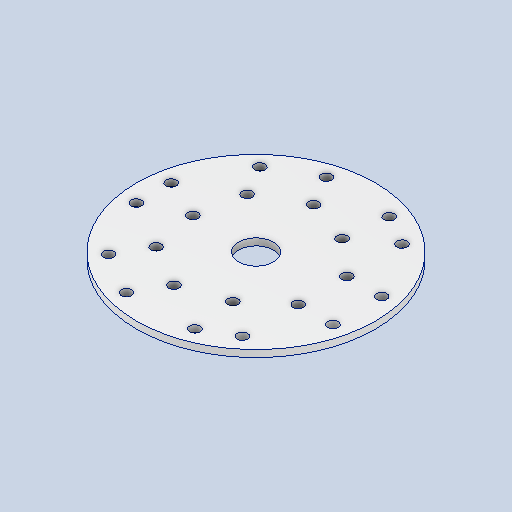
# Autodesk Inventor part: hand-grab-v1-MDF-air-Base
Saved by Autodesk Inventor 2025.1 (Build 291241000, 241)
## iProperties
Created: 2024-10-07
Part Number: hand-grab-v1-MDF-air-Base
Material: アルミニウム 6061
Document SubType Name: Modeling
Designer: haruy
Density: 2.7 g/cm^3
Appearance: アルミニウム - フラット
Author: haruy
Autodesk Inventor part; units mm, degrees
ref_plane "YZ Plane" through (0, 0, 0) normal (1, 0, 0) x (0, 1, 0)
ref_plane "XZ Plane" through (0, 0, 0) normal (0, 1, 0) x (-1, 0, 0)
ref_plane "XY Plane" through (0, 0, 0) normal (0, 0, 1) x (1, 0, 0)
derived "hand-grab-v1-Sketch-Base.ipt"
sketch "スケッチ1" plane through (400, 0, 0) normal (1, 0, 0) x (0, 1, 0)
  circle A0 centre (0, 0) radius 120
  circle A1 centre (-109.5522, 63.25) radius 6.5
  line L0 (0, 0) -> (-109.5522, 63.25)
  line L1 (0, 0) -> (0, 120)
  line L2 (246.0862, 200) -> (-251.4603, 200)
  circle A2 centre (145, 60) radius 254.573
  circle A3 centre (-67.6203, 200) radius 6.5
  line L3 (0, 0) -> (-120, 0)
  line L4 (249, 9.15) -> (187, 9.15)
  line L5 (187, 9.15) -> (187, -9.15)
  line L6 (187, -9.15) -> (249, -9.15)
  line L7 (249, -9.15) -> (249, 9.15)
  line L8 (187, 5.15) -> (179, 5.15)
  line L9 (179, 5.15) -> (179, -4.85)
  line L10 (179, -4.85) -> (187, -4.85)
  line L11 (187, -4.85) -> (187, 5.15)
  line L12 (179, 3.15) -> (174, 3.15)
  line L13 (174, 3.15) -> (174, -2.85)
  line L14 (174, -2.85) -> (179, -2.85)
  line L15 (179, -2.85) -> (179, 3.15)
  line L16 (174, 2.65) -> (159, 2.65)
  line L17 (159, 2.65) -> (159, -2.35)
  line L18 (159, -2.35) -> (174, -2.35)
  line L19 (174, -2.35) -> (174, 2.65)
  line L20 (187, 34.15) -> (184, 34.15)
  line L21 (184, 34.15) -> (184, -43.5182)
  line L22 (184, -43.5182) -> (187, -43.5182)
  line L23 (187, -43.5182) -> (187, 34.15)
  circle A4 centre (150, 65) radius 4
  circle A5 centre (150, 65) radius 14
  line L24 (187, 34.15) -> (192, 34.15)
  line L25 (192, 34.15) -> (192, 14.15)
  line L26 (192, 14.15) -> (187, 14.15)
  line L27 (187, 14.15) -> (187, 34.15)
  line L28 (184, 34.15) -> (147.5804, 61.8148)
  line L29 (151.3533, 68.7641) -> (192, 54.15)
  line L30 (192, 54.15) -> (192, 34.15)
  line L31 (239.3868, 130) -> (-239.3868, 130)
  circle A6 centre (-109.5522, 63.25) radius 4
  circle A7 centre (150, 65) radius 9
  line L32 (-106.0881, 61.25) -> (-113.0163, 65.25)
  line L33 (170, 36) -> (155, 36)
  circle A8 centre (155, 36) radius 5
  circle A9 centre (155, 36) radius 9
  circle A10 centre (-90.698, 156.1969) radius 6.5
  circle A11 centre (170, 36) radius 5
  line L34 (150, 65) -> (170, 36)
  circle A12 centre (170, 36) radius 9
  circle A13 centre (150, 65) radius 44.2278
  line L35 (150, 65) -> (155, 36)
  line L36 (150, 65) -> (-109.5522, 63.25)
  line L37 (-90.698, 156.1969) -> (150, 65)
  line L38 (150, 65) -> (157.5146, 21.4152)
  circle A14 centre (150, 65) radius 35.2278
  circle A15 centre (155.9855, 30.2844) radius 9
  line L39 (168.0777, 21.2844) -> (136, 21.2844)
  line L40 (175, 3.15) -> (175, -2.85)
  point P0 (-60, 0)
sketch "スケッチ2" plane through (0, 400, 0) normal (0, 1, 0) x (-1, 0, 0)
  circle A0 centre (0, 0) radius 120
  line L0 (0, 0) -> (-331.4625, 0) construction
  line L1 (67.5, -116.9134) -> (-135, 0)
  circle A1 centre (0, 0) radius 5
  line L2 (0, 0) -> (67.5, 116.9134) construction
  line L3 (0, 0) -> (67.5, -116.9134) construction
  line L4 (0, 0) -> (-135, 0)
  line L5 (17.0359, 37.507) -> (12.0359, 28.8468) construction
  line L6 (12.0359, 28.8468) -> (15.5, 26.8468) construction
  line L7 (15.5, 26.8468) -> (20.5, 35.507) construction
  line L8 (20.5, 35.507) -> (17.0359, 37.507)
  line L9 (20.5, 35.507) -> (15.5, 26.8468) construction
  line L10 (15.5, 26.8468) -> (18.9641, 24.8468) construction
  line L11 (18.9641, 24.8468) -> (23.9641, 33.507) construction
  line L12 (23.9641, 33.507) -> (20.5, 35.507)
  line L13 (14.5359, 33.1769) -> (21.4641, 29.1769) construction
  circle A2 centre (0, 0) radius 2.65 construction
  line L14 (16.8194, 37.632) -> (10.3194, 26.3737) construction
  line L15 (10.3194, 26.3737) -> (5.9893, 28.8737) construction
  line L16 (5.9893, 28.8737) -> (12.4893, 40.132) construction
  line L17 (12.4893, 40.132) -> (16.8194, 37.632)
  line L18 (28.5107, 30.882) -> (24.1806, 33.382)
  line L19 (22.0107, 19.6237) -> (28.5107, 30.882) construction
  line L20 (24.1806, 33.382) -> (17.6806, 22.1237) construction
  line L21 (17.6806, 22.1237) -> (22.0107, 19.6237) construction
  circle A3 centre (0, 0) radius 28.3207 construction
  line L22 (-41, 9.25) -> (-41, 4.25)
  line L23 (-41, 4.25) -> (-28, 4.25) construction
  line L24 (-28, 9.25) -> (-41, 9.25) construction
  line L25 (-28, 4.25) -> (-28, 9.25)
  line L26 (-41, -4.25) -> (-28, -4.25) construction
  line L27 (-41, -9.25) -> (-41, -4.25)
  line L28 (-28, -9.25) -> (-41, -9.25) construction
  line L29 (-28, -4.25) -> (-28, -9.25)
  line L30 (12.4893, -40.132) -> (16.8194, -37.632)
  line L31 (16.8194, -37.632) -> (10.3194, -26.3737) construction
  line L32 (5.9893, -28.8737) -> (12.4893, -40.132) construction
  line L33 (10.3194, -26.3737) -> (5.9893, -28.8737) construction
  line L34 (24.1806, -33.382) -> (17.6806, -22.1237) construction
  line L35 (28.5107, -30.882) -> (24.1806, -33.382)
  line L36 (22.0107, -19.6237) -> (28.5107, -30.882) construction
  line L37 (17.6806, -22.1237) -> (22.0107, -19.6237) construction
  line L38 (5.9893, 28.8737) -> (5.373, 27.8064)
  line L39 (22.0107, 19.6237) -> (21.3945, 18.5564) construction
  line L40 (-28, 9.25) -> (-26.7675, 9.25)
  line L41 (-28, -9.25) -> (-26.7675, -9.25)
  line L42 (5.9893, -28.8737) -> (2.1934, -22.2991) construction
  line L43 (22.0107, -19.6237) -> (21.3945, -18.5564) construction
  line L44 (13.6109, 31.5748) -> (3.6109, 14.2543) construction
  line L45 (3.6109, 14.2543) -> (-1.5853, 17.2543) construction
  line L46 (-1.5853, 17.2543) -> (8.4147, 34.5748) construction
  line L47 (8.4147, 34.5748) -> (13.6109, 31.5748)
  circle A4 centre (3.5128, 20.0844) radius 1.5
  circle A5 centre (8.5128, 28.7446) radius 1.5
  circle A6 centre (20.6372, 21.7446) radius 1.5
  circle A7 centre (15.6372, 13.0844) radius 1.5
  circle A8 centre (-29.15, 7) radius 1.5
  circle A9 centre (-19.15, 7) radius 1.5
  circle A10 centre (-19.15, -7) radius 1.5
  circle A11 centre (-29.15, -7) radius 1.5
  circle A12 centre (8.5128, -28.7446) radius 1.5
  circle A13 centre (3.5128, -20.0844) radius 1.5
  circle A14 centre (15.6372, -13.0844) radius 1.5
  circle A15 centre (20.6372, -21.7446) radius 1.5
  line L48 (1.0128, 15.7543) -> (13.6109, 31.5748) construction
  circle A16 centre (0, 0) radius 34.3835
  line L49 (-8, 47) -> (-188, 47) construction
  line L50 (-188, 47) -> (-188, 32)
  line L51 (-188, 32) -> (-8, 32) construction
  line L52 (-8, 32) -> (-8, 47) construction
  circle A17 centre (-18, 39.5) radius 1.5 construction
  circle A18 centre (-28, 39.5) radius 1.5 construction
  line L53 (-34.3835, 47) -> (-34.3835, 0) construction
  line L54 (-8, 47) -> (19.3201, 28.4422) construction
  line L55 (-8, -47) -> (-188, -47) construction
  line L56 (-188, -32) -> (-8, -32) construction
  circle A19 centre (-18, -39.5) radius 1.5 construction
  circle A20 centre (-28, -39.5) radius 1.5 construction
  line L57 (-34.3835, -47) -> (-34.3835, 0) construction
  line L58 (-8, -47) -> (19.3201, -28.4422) construction
  line L59 (0, 0) -> (-17.1917, 29.777)
  line L60 (-8.5315, 34.777) -> (-25.852, 24.777)
  line L61 (-25.852, 24.777) -> (-20.852, 16.1167)
  line L62 (-20.852, 16.1167) -> (-3.5315, 26.1167)
  line L63 (-3.5315, 26.1167) -> (-8.5315, 34.777)
  circle A21 centre (-10.3616, 27.9468) radius 1.5
  circle A22 centre (-19.0219, 22.9468) radius 1.5
  circle A23 centre (-19.0219, -22.9468) radius 1.5
  circle A24 centre (-10.3616, -27.9468) radius 1.5
  circle A25 centre (29.3835, -5) radius 1.5
  circle A26 centre (29.3835, 5) radius 1.5
  circle A27 centre (0, 0) radius 193.5
  line L64 (-192.8647, 15.6665) -> (82.8647, 174.859)
  line L65 (0, 0) -> (-60, 103.923)
  line L66 (0, 0) -> (0, 193.5)
  line L67 (53.3013, 7.6795) -> (-48.1987, 183.4826)
  line L68 (-48.1987, 183.4826) -> (-61.1891, 175.9826)
  line L69 (-61.1891, 175.9826) -> (40.3109, 0.1795)
  line L70 (40.3109, 0.1795) -> (53.3013, 7.6795)
  circle A28 centre (-21.9439, 123.008) radius 1.5
  circle A29 centre (-50.9439, 173.2375) radius 1.5
  circle A30 centre (-9.0667, 15.704) radius 1.5
  circle A31 centre (0, 0) radius 12.5
  circle A32 centre (-9.0667, -15.704) radius 1.5
  circle A33 centre (18.1335, 0) radius 1.5
  circle A34 centre (41.8061, 12.5897) radius 1.5
  circle A35 centre (31.8061, 29.9103) radius 1.5
  circle A36 centre (0, 0) radius 24.3835
  line L71 (53.3013, 7.6795) -> (22.0795, -10.3464)
  line L72 (33.3013, 42.3205) -> (2.0795, 24.2946)
  line L73 (-33.3013, -42.3205) -> (-134.8013, 133.4826)
  line L74 (-20.3109, -34.8205) -> (-33.3013, -42.3205)
  circle A37 centre (-31.8061, -29.9103) radius 1.5
  circle A38 centre (-41.8061, -12.5897) radius 1.5
  line L75 (-33.3013, -42.3205) -> (-2.0795, -24.2946)
  line L76 (-53.3013, -7.6795) -> (-22.0795, 10.3464)
  point P0 (19.3201, -28.4422)
  dimension "d3" = 3
  dimension "d4" = 3
  dimension "d5" = 10
  dimension "d6" = 10
  dimension "d7" = 7.5
  dimension "d8" = 7.5
  dimension "d10" = 60
  dimension "d12" = 10
  dimension "d13" = 10
  dimension "d14" = 10
  dimension "d15" = 3
  dimension "d17" = 5
  dimension "d18" = 5
  dimension "d21" = 360
  dimension "d25" = 387
  dimension "d26" = 110
  dimension "d27" = 60
  dimension "d28" = 15
  dimension "d30" = 73
  dimension "d31" = 3
  dimension "d32" = 3
  dimension "d33" = 7.5
  dimension "d34" = 7.5
  dimension "d35" = 7.5
  dimension "d36" = 7.5
  dimension "d37" = 3
  dimension "d38" = 25
  dimension "d39" = 6.25
  dimension "d42" = 360
  dimension "d44" = 20
  dimension "d45" = 3
  dimension "d46" = 3
  dimension "d47" = 10
  dimension "d48" = 7.5
  dimension "d49" = 7.5
  dimension "d50" = 20
  dimension "d51" = 35
  dimension "d52" = 10
  measures "d3" diameter of A17
  measures "d4" diameter of A18
  measures "d5" distance from line of A17.centre L52
  measures "d6" distance of A18.centre A17.centre
  measures "d7" distance from line of A17.centre L49
  measures "d8" distance from line of L49 A18.centre
  measures "d12" distance between parallel lines of L60 L62
  measures "d13" distance between parallel lines of L63 L59
  measures "d14" distance between parallel lines of L59 L61
  measures "d15" diameter of A21
  measures "d17" distance from line of L59 A21.centre
  measures "d18" distance from line of A21.centre L60
  measures "d25" diameter of A27
  measures "d26" distance from line of L64 A3.centre
  measures "d28" distance of L68.end L67.end
  measures "d30" distance between parallel lines of L64 L68
  measures "d31" diameter of A28
  measures "d32" diameter of A29
  measures "d33" distance from line of A28.centre L64
  measures "d34" distance from line of A28.centre L69
  measures "d35" distance from line of A29.centre L68
  measures "d36" distance from line of A29.centre L67
  measures "d37" diameter of A30
  measures "d38" diameter of A31
  measures "d39" distance from line of A30.centre L62
  measures "d44" distance from line of L70 point (0, 0)
  measures "d45" diameter of A34
  measures "d46" diameter of A35
  measures "d47" distance from line of A34.centre L70
  measures "d48" distance from line of L67 A35.centre
  measures "d49" distance from line of L67 A34.centre
  measures "d50" distance of A35.centre A34.centre
  measures "d51" distance from line of L69 point (0, 0)
  measures "d52" distance from line of L72 A35.centre
ref_plane "作業平面1" through (400, 0, 0) normal (1, 0, 0) x (0, 1, 0)
ref_plane "作業平面2" through (0, 400, 0) normal (0, 1, 0) x (-1, 0, 0)
extrude "押し出し1" add sketch "スケッチ2" along normal blind 2 contours L66 A36 L62 L63 A16 | A16 L72 A5 A36 L66 | L63 L62 L59 A16 | A36 L4 A31 L66 | L66 A31 L59 A30 A36 | L59 L62 L61 A16 | A16 L71 A25 A36 L72 A5 | A31 L4 A1 L66 | L66 A1 L59 A31 | A36 L76 A8 A16 L61 L62 | L59 A30 A31 L4 A36 | A16 L75 A24 A36 L71 A25 | A16 L76 A8 A36 L4 | L4 A36 L75 A24 A16 | L59 A1 L4 A31
sketch "スケッチ3" plane through (0, 402, 0) normal (0, 1, 0) x (0, 0, -1)
  circle A0 centre (0, 0) radius 34.3835 projected
  circle A1 centre (0, 0) radius 5 projected
  circle A2 centre (21.7446, 20.6372) radius 1.5 projected
  circle A3 centre (13.0844, 15.6372) radius 1.5 projected
  circle A4 centre (20.0844, 3.5128) radius 1.5 projected
  circle A5 centre (28.7446, 8.5128) radius 1.5 projected
  circle A6 centre (7, -29.15) radius 1.5 projected
  circle A7 centre (7, -19.15) radius 1.5 projected
  circle A8 centre (-7, -19.15) radius 1.5 projected
  circle A9 centre (-7, -29.15) radius 1.5 projected
  circle A10 centre (-21.7446, 20.6372) radius 1.5 projected
  circle A11 centre (-13.0844, 15.6372) radius 1.5 projected
  circle A12 centre (-28.7446, 8.5128) radius 1.5 projected
  circle A13 centre (-20.0844, 3.5128) radius 1.5 projected
sketch "スケッチ4" plane through (0, 402, 0) normal (0, 1, 0) x (1, 0, 0)
  circle A0 centre (0, 0) radius 34.3835 projected
  circle A1 centre (0, 0) radius 5 projected
  circle A2 centre (19.15, -7) radius 1.5 projected
  circle A3 centre (10.3616, 27.9468) radius 1.5 projected
  circle A4 centre (29.15, 7) radius 1.5 projected
  circle A5 centre (19.0219, 22.9468) radius 1.5 projected
  circle A6 centre (-8.5128, 28.7446) radius 1.5 projected
  circle A7 centre (-20.6372, 21.7446) radius 1.5 projected
  circle A8 centre (29.15, -7) radius 1.5 projected
  circle A9 centre (-18.1335, 0) radius 1.5 projected
  circle A10 centre (9.0667, 15.704) radius 1.5 projected
  circle A11 centre (-15.6372, 13.0844) radius 1.5 projected
  circle A12 centre (-3.5128, 20.0844) radius 1.5 projected
  circle A13 centre (19.15, 7) radius 1.5 projected
  circle A14 centre (-15.6372, -13.0844) radius 1.5 projected
  circle A15 centre (-3.5128, -20.0844) radius 1.5 projected
  circle A16 centre (-8.5128, -28.7446) radius 1.5 projected
  circle A17 centre (-20.6372, -21.7446) radius 1.5 projected
  circle A18 centre (-29.3835, -5) radius 1.5 projected
  circle A19 centre (-29.3835, 5) radius 1.5 projected
  circle A20 centre (9.0667, -15.704) radius 1.5 projected
  circle A21 centre (10.3616, -27.9468) radius 1.5 projected
  circle A22 centre (19.0219, -22.9468) radius 1.5 projected
equation "\"d8\" = d7"
